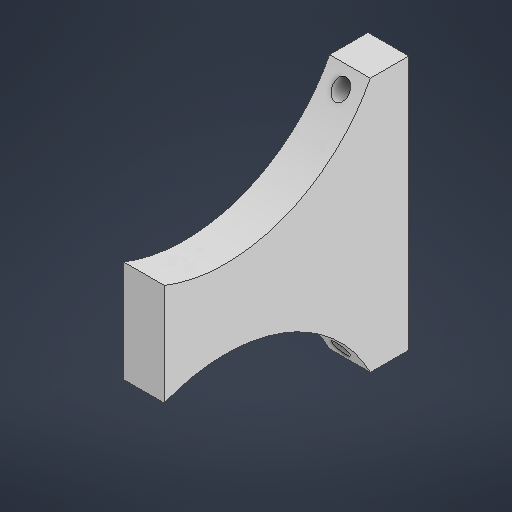
# Autodesk Inventor part: Caliper Bracket Mount V2
Saved by Autodesk Inventor 2026.1 (Build 301233000, 233)
## iProperties
Created: 2026-06-29
Part Number: Caliper Bracket Mount V2
Material: Generic
Document SubType Name: Modeling
Designer: share
Density: 1 g/cm^3
Appearance: Default
Author: share
Autodesk Inventor part; units mm, degrees
ref_plane "YZ Plane" through (0, 0, 0) normal (1, 0, 0) x (0, 1, 0)
ref_plane "XZ Plane" through (0, 0, 0) normal (0, 1, 0) x (-1, 0, 0)
ref_plane "XY Plane" through (0, 0, 0) normal (0, 0, 1) x (1, 0, 0)
sketch "Sketch1" plane through (0, 0, 0) normal (1, 0, 0) x (0, 1, 0)
  line L0 (0, 144) -> (0, -24) construction
  line L1 (-138.8268, 0) -> (138.8268, 0) construction
  line L2 (-62.5, 0) -> (-62.5, 18.8952)
  line L3 (62.5, 0) -> (62.5, 18.8952)
  line L4 (25, 120) -> (-25, 120)
  line L5 (62.5, 0) -> (-62.5, 0)
  arc A0 (25, 120) -> (62.5, 18.8952) centre (99.162, 90) ccw
  arc A1 (-62.5, 18.8952) -> (-25, 120) centre (-99.162, 90) ccw
  point P0 (0, 0)
  dimension "d0" = 120
  dimension "d1" = 125
  dimension "d3" = 50
  dimension "d4" = 80
  dimension "d6" = 90
  constraints: 8 end point, 4 point on circle, 4 symmetric about line, 2 centre point, 1 parallel, 1 point on line, 1 vertical, 1 other
  measures "d0" distance between parallel lines of L1 L4
  measures "d1" distance between parallel lines of L2 L3
  measures "d3" distance of L4.start L4.end
  measures "d4" radius of A0
  measures "d6" distance from line of L5 A0.centre
extrude "Main Body" add sketch "Sketch1" along normal mid plane 20
sketch "Sketch2" plane through (10, 62.5, 0) normal (0, 0, -1) x (-1, 0, 0)
  line L0 (20, 0) -> (0, 0) projected
  line L1 (10, 0) -> (10, -125) construction
  line L2 (20, -125) -> (0, -125) projected
  line L3 (0, -37.5) -> (0, -87.5) projected
  line L4 (0, -62.5) -> (20, -62.5) construction
  line L5 (20, -87.5) -> (20, -37.5) projected
  circle A0 centre (10, -7.5) radius 4
  circle A1 centre (10, -117.5) radius 4
  point P0 (10, -62.5)
  dimension "d9" = 110
  dimension "d10" = 8
  constraints: 4 end point, 4 midpoint, 2 centre point, 1 point on line, 1 symmetric about line, 1 other
  measures "d9" distance of A1.centre A0.centre
  measures "d10" diameter of A0
extrude "Upright Mount Holes" cut sketch "Sketch2" against normal through all
sketch "Sketch3" plane through (-10, 0, 0) normal (-1, 0, 0) x (0, 0, 1)
  line L0 (0, 87.5) -> (0, -87.5) construction
  line L1 (-24, 0) -> (144, 0) construction
  circle A0 centre (10.5903, 5) radius 5
  circle A1 centre (95, -5) radius 5
  line L2 (10.5903, 5) -> (95, -5) construction
  circle A2 centre (10.5903, 5) radius 2.5
  circle A3 centre (95, -5) radius 2.5
  point P0 (0, 0)
  dimension "d13" = 5
  dimension "d14" = 5
  dimension "d15" = 95
  dimension "d16" = 85
  dimension "d17" = 10
  dimension "d18" = 5
  constraints: 4 centre point, 2 coincident, 2 end point, 2 equal radius
  measures "d13" distance from line of L2.end L1
  measures "d14" distance from line of L1 L2.start
  measures "d15" distance from line of L0 L2.end
  measures "d16" distance of L2.start L2.end
  measures "d17" diameter of A0
  measures "d18" diameter of A3
extrude "Extrusion3" add sketch "Sketch3" along normal blind 10
body "Solid1"
